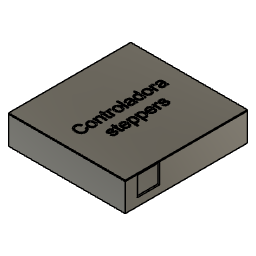
controladora sttepers (v1~recovered) (Autodesk Fusion 360 design; units mm, degrees)
Autodesk Fusion 360 part; units mm, degrees
sketch "Sketch1" plane through (0, 0, 0) normal (0, 0, 1) x (1, 0, 0)
  line L0 (0, 0) -> (105, 0)
  line L1 (105, 0) -> (105, 110)
  line L2 (105, 110) -> (0, 110)
  line L3 (0, 110) -> (0, 0)
  dimension "d1" = 105
  dimension "d2" = 110
  constraint horizontal L0
  constraint vertical L1
  constraint horizontal L2
  constraint vertical L3
  constraint coincident L0.start L3.end
  measures "d1" distance of L0.start L0.end
  measures "d2" distance of L0.start L2.end
extrude "Extrude1" add sketch "Sketch1" along normal blind 25 makes body 1
shell "Shell1" thickness 1.5 removed faces 1 at (35, 73.3333, 25) on bodies 1
sketch "Sketch2" plane through (0, 0, 1.5) normal (0, 0, 1) x (-1, 0, 0)
  line L0 (-1.5, -108.5) -> (-1.5, -1.5)
  line L1 (-1.5, -1.5) -> (-103.5, -1.5)
  line L2 (-103.5, -1.5) -> (-103.5, -108.5)
  line L3 (-103.5, -108.5) -> (-1.5, -108.5)
  line L4 (-1.5, -108.5) -> (-6.5, -108.5)
  line L5 (-1.5, -108.5) -> (-1.5, -103.5)
  circle A0 centre (-6.5, -103.5) radius 1.75
  line L6 (-103.5, -108.5) -> (-98.5, -108.5)
  line L7 (-103.5, -108.5) -> (-103.5, -103.5)
  circle A1 centre (-98.5, -103.5) radius 1.75
  line L8 (-103.5, -1.5) -> (-103.5, -6.5)
  line L9 (-103.5, -1.5) -> (-98.5, -1.5)
  circle A2 centre (-98.5, -6.5) radius 1.75
  line L10 (-1.5, -1.5) -> (-1.5, -6.5)
  line L11 (-1.5, -1.5) -> (-6.5, -1.5)
  circle A3 centre (-6.5, -6.5) radius 1.75
  dimension "d6" = 5
  dimension "d7" = 5
  dimension "d8" = 3.5
  dimension "d9" = 5
  dimension "d10" = 5
  dimension "d11" = 3.5
  dimension "d12" = 5
  dimension "d13" = 5
  dimension "d14" = 3.5
  dimension "d15" = 5
  dimension "d16" = 5
  dimension "d17" = 3.5
  constraint coincident L0.start L3.end
  constraint perpendicular L0 L4
  constraint perpendicular L3 L5
  constraint coincident L2.end L3.start
  constraint perpendicular L2 L6
  constraint perpendicular L6 L7
  constraint coincident L1.end L2.start
  constraint perpendicular L1 L8
  constraint perpendicular L8 L9
  constraint coincident L0.end L1.start
  constraint perpendicular L1 L10
  constraint perpendicular L0 L11
  measures "d6" distance of L0.start L4.end
  measures "d7" distance of L0.start L5.end
  measures "d8" diameter of A0
  measures "d9" distance of L2.end L6.end
  measures "d10" distance of L2.end L7.end
  measures "d11" diameter of A1
  measures "d12" distance of L1.end L8.end
  measures "d13" distance of L1.end L9.end
  measures "d14" diameter of A2
  measures "d15" distance of L0.end L10.end
  measures "d16" distance of L0.end L11.end
  measures "d17" diameter of A3
extrude "Extrude2" cut sketch "Sketch2" against normal blind 35 contours A0 | A1 | A2 | A3 bodies 1
sketch "Sketch3" plane through (0, 110, 0) normal (0, 1, 0) x (-1, 0, 0)
  line L0 (-105, 0) -> (0, 0)
  line L1 (0, 0) -> (0, 25)
  line L2 (0, 25) -> (-105, 25)
  line L3 (-105, 25) -> (-105, 0)
  line L4 (-105, 25) -> (-85, 25)
  line L5 (0, 25) -> (-20, 25)
  line L6 (-85, 25) -> (-85, 7)
  line L7 (-85, 7) -> (-20, 7)
  line L8 (-20, 7) -> (-20, 25)
  dimension "d20" = 20
  dimension "d21" = 20
  dimension "d22" = 18
  constraint coincident L2.end L3.start
  constraint perpendicular L3 L4
  constraint coincident L1.end L2.start
  constraint perpendicular L1 L5
  constraint perpendicular L2 L6
  constraint perpendicular L6 L7
  constraint perpendicular L5 L8
  measures "d20" distance of L2.end L4.end
  measures "d21" distance of L1.end L5.end
  measures "d22" distance of L4.end L6.end
extrude "Extrude3" cut sketch "Sketch3" against normal blind 20 contours L2 L6 L7 L8 bodies 1
sketch "Sketch4" plane through (105, 0, 0) normal (1, 0, 0) x (0, 1, 0)
  line L0 (0, 0) -> (110, 0)
  line L1 (110, 0) -> (110, 25)
  line L2 (110, 25) -> (0, 25)
  line L3 (0, 25) -> (0, 0)
  line L4 (1, 25) -> (11, 25)
  line L5 (11, 25) -> (11, 7)
  line L6 (11, 7) -> (31, 7)
  line L7 (31, 7) -> (31, 25)
  dimension "d25" = 10
  dimension "d26" = 18
  dimension "d27" = 20
  constraint coincident L2 L4.start
  constraint perpendicular L3 L4
  constraint perpendicular L2 L5
  constraint perpendicular L5 L6
  constraint coincident L2 L7.end
  constraint perpendicular L2 L7
  measures "d25" distance of L4.start L4.end
  measures "d26" distance of L4.end L5.end
  measures "d27" distance of L5.end L6.end
extrude "Extrude4" cut sketch "Sketch4" against normal blind 170 contours L2 L5 L6 L7 bodies 1
sketch "Sketch5" plane through (0, 0, 0) normal (0, 0, 1) x (1, 0, 0)
  line L0 (105, 0) -> (0, 0)
  line L1 (0, 0) -> (0, 110)
  line L2 (0, 110) -> (105, 110)
  line L3 (105, 110) -> (105, 0)
  constraint horizontal L0
  constraint vertical L1
  constraint horizontal L2
  constraint vertical L3
extrude "Extrude5" add sketch "Sketch5" along normal blind 1 separate body makes body 2
move_body "Move1" bodies 2 to x (1, 0, 0) y (0, 1, 0) z (0, 0, 1) at (0, 0, 25)
sketch "Sketch6" plane through (0, 0, 25) normal (0, 0, -1) x (1, 0, 0)
  line L0 (0, -110) -> (105, -110)
  line L1 (105, -110) -> (105, 0)
  line L2 (105, 0) -> (0, 0)
  line L3 (0, 0) -> (0, -110)
  line L4 (105, -110) -> (103.5, -110)
  line L5 (103.5, -110) -> (103.5, -108.5)
  line L6 (0, -110) -> (1.5, -110)
  line L7 (0, -110) -> (0, -108.5)
  line L8 (0, 0) -> (0, -1.5)
  line L9 (0, 0) -> (1.5, 0)
  line L10 (105, 0) -> (105, -1.5)
  line L11 (105, 0) -> (103.5, 0)
  line L12 (103.5, -1.5) -> (1.5, -1.5)
  line L13 (1.5, -1.5) -> (1.5, -108.5)
  line L14 (1.5, -108.5) -> (103.5, -108.5)
  line L15 (103.5, -108.5) -> (103.5, -1.5)
  dimension "d32" = 1.5
  dimension "d33" = 1.5
  dimension "d34" = 1.5
  dimension "d35" = 1.5
  dimension "d36" = 1.5
  dimension "d37" = 1.5
  dimension "d38" = 1.5
  dimension "d39" = 1.5
  constraint coincident L0.end L1.start
  constraint perpendicular L1 L4
  constraint perpendicular L4 L5
  constraint coincident L0.start L3.end
  constraint perpendicular L3 L6
  constraint perpendicular L6 L7
  constraint coincident L2.end L3.start
  constraint perpendicular L2 L8
  constraint perpendicular L3 L9
  constraint coincident L1.end L2.start
  constraint vertical L10
  constraint horizontal L11
  constraint horizontal L12
  constraint vertical L13
  constraint horizontal L14
  constraint vertical L15
  measures "d32" distance of L0.end L4.end
  measures "d33" distance of L4.end L5.end
  measures "d34" distance of L0.start L6.end
  measures "d35" distance of L0.start L7.end
  measures "d36" distance of L2.end L8.end
  measures "d37" distance of L2.end L9.end
  measures "d38" distance of L1.end L10.end
  measures "d39" distance of L1.end L11.end
extrude "Extrude6" add sketch "Sketch6" along normal blind 2 contours L12 L13 L14 L15 bodies 2
sketch "Sketch7" plane through (0, 0, 26) normal (0, 0, 1) x (-1, 0, 0)
  line L0 (-105, -110) -> (0, -110)
  line L1 (0, -110) -> (0, 0)
  line L2 (0, 0) -> (-105, 0)
  line L3 (-105, 0) -> (-105, -110)
  line L4 (-105, 0) -> (-105, -110) construction
  line L5 (-105, -110) -> (0, -110) construction
  line L6 (0, -110) -> (0, 0) construction
  line L7 (0, 0) -> (-105, 0) construction
  dimension "d42" = 10
  text T0 "Controladora \nsteppers " font "Arial" height 10 align centre middle in box 110 x 105 at (-105, 0) x (0, -1) y (1, 0) spacing 1
  constraint coincident L0.start
  constraint coincident L1.end
extrude "Extrude7" cut sketch "Sketch7" against normal blind 2 text T0 bodies 2
